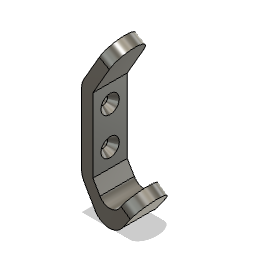
Coat Hook v4 (Autodesk Fusion 360 design; units mm, degrees)
Autodesk Fusion 360 part; units mm, degrees
sketch "Sketch1" plane through (0, 0, 0) normal (0, 0, 1) x (1, 0, 0)
  line L0 (11.5304, 55) -> (-0.0094, 35)
  line L1 (-0.0094, 35) -> (0, 0)
  line L2 (0, 0) -> (6.0773, -10.5197)
  line L3 (17.8607, -11.0501) -> (25.6471, 0)
  line L4 (15.8612, 52.5012) -> (4.9909, 33.6616)
  line L5 (4.9909, 33.6616) -> (4.9996, 1.3411)
  line L6 (4.9996, 1.3411) -> (8.0596, -3.9556)
  line L7 (16.4762, -4.3344) -> (21.5599, 2.88)
  line L8 (11.5304, 55) -> (15.8612, 52.5012)
  line L9 (25.6471, 0) -> (21.5599, 2.88)
  arc A0 (8.0596, -3.9556) -> (16.4762, -4.3344) centre (12.389, -1.4544) ccw
  arc A1 (6.0773, -10.5197) -> (17.8607, -11.0501) centre (12.1386, -7.0181) ccw
  point P0 (11.5542, -20)
  dimension "d16" = 35
  dimension "d17" = 150
  dimension "d18" = 150
  dimension "d19" = 20
  dimension "d20" = 20
  dimension "d21" = 20
  dimension "d23" = 5
  dimension "d24" = 7
  constraint coincident L1.end L2.start
  constraint perpendicular L3 L9
  constraint parallel L0 L4
  constraint parallel L1 L5
  constraint parallel L2 L6
  constraint parallel L3 L7
  constraint tangent L6 A0
  constraint tangent L7 A0
  constraint coincident P0 L2
  constraint coincident P0 L3
  constraint tangent L2 A1
  constraint tangent L3 A1
  measures "d16" vertical distance of L0.end L1.end
  measures "d17" angle of L0 L1
  measures "d18" angle of L1 L2
  measures "d19" vertical distance of L0.start L0.end
  measures "d20" vertical distance of P0 L3.end
  measures "d21" vertical distance of L1.end P0
  measures "d23" radius of A0
  measures "d24" radius of A1
extrude "Extrude1" add sketch "Sketch1" along normal blind 15
sketch "Sketch2" plane through (5, 0.0013, 0) normal (1, 0.00027, 0) x (0, 0, -1)
  line L0 (0, 1.3397) -> (0, 33.6603)
  line L1 (0, 33.6603) -> (-15, 33.6603)
  line L2 (-15, 33.6603) -> (-15, 1.3397)
  line L3 (-15, 1.3397) -> (0, 1.3397)
  line L4 (-7.5, 33.6603) -> (-7.5, 1.3397) construction
  line L5 (0, 17.5) -> (-15, 17.5) construction
  circle A0 centre (-7.5, 25.6603) radius 4
  circle A1 centre (-7.5, 9.3397) radius 4
  dimension "d27" = 8
  dimension "d28" = 8
  constraint midpoint L1 L4.start
  constraint midpoint L3 L4.end
  constraint midpoint L0 L5.start
  constraint midpoint L2 L5.end
  constraint coincident L4 A0.centre
  constraint symmetric L5 A0 A1
  measures "d27" diameter of A0
  measures "d28" distance of L1 A0.centre
extrude "Extrude2" cut sketch "Sketch2" against normal blind 3 draft -35 contours A0 | A1
extrude "Extrude3" cut 2 faces at (1.9929, 26.1558, 7.387) (1.9973, 9.8353, 7.0106) along direction (-1, -0.00027, 0) through all
fillet "Fillet1" radius 7.5 4 edges at (13.6958, 53.7506, 15) (13.6958, 53.7506, 0) (23.6035, 1.44, 15) (23.6035, 1.44, 0)
fillet "Fillet2" radius 8 2 edges at (-0.0094, 35, 7.5) (0, 0, 7.5)
